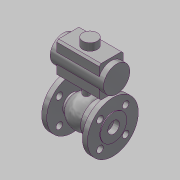
# Autodesk Inventor part: BALL VALVE  PNEUMATIC FLANGED S235 DN32
Saved by Autodesk Inventor 2017 (Build 210142000, 142)
## iProperties
Category: Piping Part
Company: Demarec
Created: 2012-12-20
Part Number: BALL VALVE  PNEUMATIC FLANGED S235 DN32
Material: S235
Document SubType Name: Modeling
Designer: Marc Crauwels
Density: 7.85 g/cm^3
Mass: 658107 g
Surface Area: 21375.3 cm^2
Volume: 83622.3 cm^3
Appearance: Steel
Description: BELVEN BV4
Author: Marc Crauwels
Title: Carbon Steel Globe Valve PN16
Comments: iPart CS GlbVlvPN16
Autodesk Inventor part; units mm, degrees
ref_plane "XZ Plane" through (0, 0, 0) normal (0, 1, 0) x (-1, 0, 0)
sketch "Sketch1" plane through (0, 0, 0) normal (1, 0, 0) x (0, 1, 0)
  line L0 (49, 16) -> (63, 16)
  line L1 (63, 16) -> (63, 70)
  line L2 (63, 70) -> (49, 70)
  line L3 (49, 70) -> (49, 16)
  line L4 (63, 16) -> (65, 16)
  line L5 (65, 16) -> (65, 36)
  line L6 (65, 36) -> (63, 36)
  line L7 (63, 36) -> (63, 16)
  line L8 (-65, 0) -> (65, 0) construction
  line L9 (65, 0) -> (49, 0) construction
  line L10 (0, 0) -> (0, 95.8184) construction
  line L11 (-65, 0) -> (-49, 0) construction
  line L12 (0, 0) -> (-21.3713, 0)
  dimension "Lenght" = 130
  dimension "DN" = 32
  dimension "FlgDia" = 140
  dimension "FlgThck" = 16
  dimension "GsktFace" = 72
  dimension "Face" = 2
  constraints: 26 end point, 5 point on line, 4 parallel, 3 horizontal, 3 perpendicular, 2 coincident, 2 collinear, 1 midpoint
  measures "Lenght" distance of L8.start L8.end
  measures "DN" diameter of L0 L8
  measures "FlgDia" diameter of L2 L8
  measures "FlgThck" distance between parallel lines of L3 L5
  measures "GsktFace" diameter of L5.end L8
  measures "Face" distance of L5.end L6.end
revolve "Revolution1" add sketch "Sketch1" angle 360 about axis through (0, -65, 0) along (0, 1, 0)
sketch "Sketch5" plane through (0, 63, 0) normal (0, 1, 0) x (1, 0, 0)
  line L0 (0, 0) -> (-35.3553, 35.3553)
  line L1 (0, 0) -> (0, 103.939) construction
  circle A0 centre (-35.3553, 35.3553) radius 9
  point P0 (0, 0)
  dimension "d16" = 50
  dimension "d17" = 45
  dimension "d18" = 18
  constraints: 4 end point, 2 coincident, 1 centre point, 1 vertical
  measures "d16" distance of L0.start L0.end
  measures "d17" angle of L1 L0
  measures "d18" diameter of A0
extrude "Extrusion2" cut sketch "Sketch5" against normal through all
pattern_circular "Circular Pattern1" count 4 over 360 about axis through (0, 64, 0) along (0, 1, 0) of "Extrusion2"
sketch "Sketch14" plane through (0, 49, 0) normal (0, -1, 0) x (-1, 0, 0)
  circle A0 centre (0, 0) radius 16 projected
  circle A1 centre (0, 0) radius 26
  dimension "d54" = 10
  constraints: 1 centre point
  measures "d54" radial gap between concentric circles of A1 A0
pattern_circular "Circular Pattern2" count 2 over 360 about axis through (-10, 0, 0) along (1, 0, 0) of "Revolution1", "Extrusion2", "Circular Pattern1"
extrude "Extrusion5" add sketch "Sketch14" along normal up to surface (98 mm away) contours A0 | A1
sketch "Sketch20" plane through (0, 0, 0) normal (1, 0, 0) x (0, 1, 0)
  line L0 (10, -42.6) -> (10, 42.6)
  arc A0 (10, -42.6) -> (10, 42.6) centre (10, 0) ccw
  line L1 (65, -37.9012) -> (65, 33.7766)
  line L2 (10, 0) -> (18.52, 0)
  line L3 (18.52, 0) -> (18.52, 76)
  line L4 (18.52, 76) -> (10, 76)
  line L5 (10, 76) -> (10, 0)
  line L6 (65, -36) -> (65, 36) projected
  point P0 (0, 0)
  point P1 (12.4178, -1.9012)
  point P2 (12.4178, -1.9012)
  point P3 (65, -37.9012)
  point P4 (0, 0)
  dimension "d78" = 85.2
  dimension "oI" = 55
  dimension "oH" = 76
  dimension "d81" = 8.52
  constraints: 10 end point, 2 parallel, 2 point on circle, 2 vertical, 1 centre point, 1 coincident, 1 horizontal, 1 midpoint, 1 perpendicular, 1 point on line, 7 other
  measures "d78" distance of L0.start L0.end
  measures "oH" distance of L4.end L2.start
  measures "d81" distance of L4.end L3.end
revolve "Revolution5" add sketch "Sketch20" angle 360 about axis through (0, 10, 76) along (0, 0, -1)
ref_plane "Work Plane1" through (0, -32.6, 0) normal (0, -1, 0) x (1, 0, 0)
sketch "Sketch21" plane through (0, -32.6, 0) normal (0, -1, 0) x (1, 0, 0)
  circle A0 centre (0, 0) radius 26 projected
  circle A1 centre (0, 0) radius 42.5
  point P0 (0, 0)
  dimension "d92" = 85
  constraints: 1 centre point, 1 coincident
  measures "d92" diameter of A1
extrude "Extrusion9" add sketch "Sketch21" against normal blind 16
ref_plane "Work Plane2" through (0, 10, 38) normal (1, 0, 0) x (0, 0, -1)
sketch "Sketch22" plane through (0, 0, 0) normal (0, 1, 0) x (-1, 0, 0)
  line L0 (33, 76) -> (-33, 76)
  line L1 (-33, 76) -> (-33, 163)
  line L2 (-33, 163) -> (33, 163)
  line L3 (33, 163) -> (33, 76)
  line L4 (0, 163) -> (20, 163)
  line L5 (20, 163) -> (20, 183)
  line L6 (20, 183) -> (0, 183)
  line L7 (0, 183) -> (0, 163)
  line L8 (33, 76) -> (-33, 163)
  circle A0 centre (0, 119.5) radius 36
  line L9 (-55.04, 76) -> (0, 76)
  line L10 (-8.52, 76) -> (8.52, 76) projected
  dimension "oCylWith" = 66
  dimension "oCylHeight" = 87
  dimension "d97" = 20
  dimension "d98" = 20
  dimension "oCylDia" = 72
  constraints: 20 end point, 4 midpoint, 4 parallel, 2 collinear, 2 perpendicular, 1 centre point
  measures "oCylWith" distance of L1.end L2.end
  measures "oCylHeight" distance of L0.end L1.end
  measures "d97" distance of L6.end L5.end
  measures "d98" distance of L5.end L4.end
  measures "oCylDia" diameter of A0
extrude "Extrusion10" add sketch "Sketch22" along normal mid plane 147 contours A0 L8 L3 | L3 A0 | A0 L1 L8 | A0 L1 picked at (11, 114.7042) picked at (-15.4028, 107.9455)
extrude "Extrusion11" add sketch "Sketch22" along normal mid plane 117 contours L8 A0 L3 | L0 L1 A0 L8 | A0 L8 L3 | A0 L1 L8 | A0 L8 L2 L3 | A0 L1 L8
revolve "Revolution6" add sketch "Sketch22" angle 360 about axis through (0, 0, 183) along (0, 0, -1) contours L2 L7 L6 L5
chamfer "Chamfer1" distance 5 angle 45 4 edges at (-33, 0, 163) (33, 0, 163) (33, 0, 76) (-33, 0, 76)
equation "\"d16\" = 0.5 * KDia"
equation "\"KDia\" = 100"
body "Solid1"
